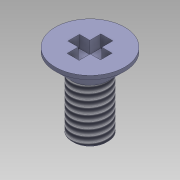
# Autodesk Inventor part: Винт М3х6 пот
Saved by Autodesk Inventor 2018 (Build 220112000, 112)
## iProperties
Created: 2020-03-17
Part Number: Винт М3х6 пот
Material: Типовые
Document SubType Name: Modeling
Designer: Leancher
Density: 1 g/cm^3
Appearance: По умолчанию
Author: Leancher
Autodesk Inventor part; units mm, degrees
ref_plane "YZ Plane" through (0, 0, 0) normal (1, 0, 0) x (0, 1, 0)
ref_plane "XZ Plane" through (0, 0, 0) normal (0, 1, 0) x (-1, 0, 0)
ref_plane "XY Plane" through (0, 0, 0) normal (0, 0, 1) x (1, 0, 0)
sketch "Эскиз1" plane through (0, 0, 0) normal (0, 1, 0) x (-1, 0, 0)
  line L0 (0, 0) -> (-2.8, 0)
  line L1 (0, 0) -> (0, -6)
  line L2 (0, -6) -> (-1.3212, -6)
  line L3 (-1.45, -5.8712) -> (-1.45, -1.65)
  line L4 (-2.8, -0.3) -> (-1.45, -1.65)
  line L5 (-2.8, 0) -> (-2.8, -0.3)
  line L6 (-1.45, -5.8712) -> (-1.3212, -6)
  constraints: 14 end point, 2 perpendicular, 1 horizontal, 1 vertical
revolve "Вращение1" add sketch "Эскиз1" angle 360 about axis through (0, 0, 0) along (0, 0, -1)
sketch "Эскиз2" plane through (0, 0, 0) normal (0, 0, 1) x (1, 0, 0)
  line L0 (-1.3212, -0.4705) -> (-1.3212, 0.4705)
  line L1 (1.3212, 0.4705) -> (1.3212, -0.4705)
  circle A0 centre (0, 0) radius 1.45 projected
  line L2 (0.4865, -1.366) -> (-0.4865, -1.366)
  line L3 (-0.4865, 1.366) -> (0.4865, 1.366)
  line L4 (1.3212, -0.4705) -> (0.4865, -0.4705)
  line L5 (-0.4865, -0.4705) -> (-1.3212, -0.4705)
  line L6 (-0.4865, -1.366) -> (-0.4865, -0.4705)
  line L7 (-0.4865, 0.4705) -> (-0.4865, 1.366)
  line L8 (-1.3212, 0.4705) -> (-0.4865, 0.4705)
  line L9 (0.4865, 0.4705) -> (1.3212, 0.4705)
  line L10 (0.4865, 1.366) -> (0.4865, 0.4705)
  line L11 (0.4865, -0.4705) -> (0.4865, -1.366)
  constraints: 24 end point, 10 parallel, 4 perpendicular, 3 horizontal, 1 point on circle
extrude "Выдавливание1" cut sketch "Эскиз2" against normal blind 1 contours L0 L8 L7 L3 L10 L9 L1 L4 L11 L2 L6 L5
thread "Резьба1" size "M3x0.5" class "6g" standard "ANSI Metric M Profile" full length
